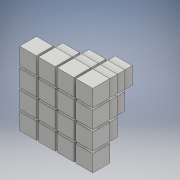
# Autodesk Inventor part: 方塊
Saved by Autodesk Inventor 2017 (Build 210142000, 142)
## iProperties
Created: 2021-05-20
Part Number: 方塊
Material: Generic
Document SubType Name: Modeling
Designer: user
Density: 1 g/cm^3
Appearance: Default
Author: user
Autodesk Inventor part; units mm, degrees
ref_plane "YZ Plane" through (0, 0, 0) normal (1, 0, 0) x (0, 1, 0)
ref_plane "XZ Plane" through (0, 0, 0) normal (0, 1, 0) x (-1, 0, 0)
ref_plane "XY Plane" through (0, 0, 0) normal (0, 0, 1) x (1, 0, 0)
sketch "Sketch1" plane through (0, 0, 0) normal (0, 1, 0) x (-1, 0, 0)
  line L0 (0, 0) -> (90, 0)
  line L1 (90, 0) -> (90, -90)
  line L2 (90, -90) -> (0, -90)
  line L3 (0, -90) -> (0, 0)
  dimension "d0" = 90
  dimension "d1" = 90
  constraints: 8 end point, 2 parallel, 1 horizontal, 1 perpendicular
  measures "d0" distance of L0.start L0.end
  measures "d1" distance of L2.end L0.start
extrude "Extrusion1" add sketch "Sketch1" along normal blind 90
pattern_linear "Rectangular Pattern1" count 4 spacing 100 along (0, 0, -1) count 4 spacing 100 along (1, 0, 0)
sketch "Sketch2" plane through (0, 90, 0) normal (0, 1, 0) x (1, 0, 0)
  line L0 (-40, 50) -> (50, 50)
  line L1 (50, 50) -> (50, 140)
  line L2 (50, 140) -> (-40, 140)
  line L3 (-40, 140) -> (-40, 50)
  line L4 (10, 100) -> (100, 100) projected
  line L5 (0, 0) -> (0, 90) projected
  line L6 (10, 100) -> (0, 90)
  point P0 (5, 95)
  dimension "d10" = 45
  dimension "d11" = 45
  dimension "d12" = 90
  dimension "d13" = 90
  constraints: 10 end point, 2 parallel, 1 horizontal, 1 midpoint, 1 perpendicular
  measures "d10" distance from line of L3 point (5, 95)
  measures "d11" distance from line of L0 point (5, 95)
  measures "d12" distance of L1.end L2.end
  measures "d13" distance of L2.end L0.start
extrude "Extrusion2" add sketch "Sketch2" along normal blind 90 separate body
pattern_linear "Rectangular Pattern2" count 3 spacing 100 along (1, 0, 0) count 3 spacing 100 along (0, 0, -1) bodies 2
sketch "Sketch3" plane through (0, 180, 0) normal (0, 1, 0) x (1, 0, 0)
  line L0 (10, 100) -> (100, 100) projected
  line L1 (100, 100) -> (100, 190) projected
  line L2 (100, 190) -> (10, 190) projected
  line L3 (10, 190) -> (10, 100) projected
  point P0 (0, 0)
extrude "Extrusion3" add sketch "Sketch3" along normal blind 90 separate body
pattern_linear "Rectangular Pattern3" count 2 spacing 100 along (0, 0, -1) count 2 spacing 100 along (1, 0, 0) bodies 3
sketch "Sketch4" plane through (10, 270, -200) normal (0, 1, 0) x (1, 0, 0)
  line L0 (50, -50) -> (140, -50) projected
  line L1 (140, -50) -> (140, 40) projected
  line L2 (140, 40) -> (50, 40) projected
  line L3 (50, 40) -> (50, -50) projected
  point P0 (-10, -200)
extrude "Extrusion4" add sketch "Sketch4" along normal blind 90 separate body
body "Solid1"
body "Solid2"
body "Solid3"
body "Solid4"
body "Solid5"
body "Solid6"
body "Solid7"
body "Solid8"
body "Solid9"
body "Solid10"
body "Solid11"
body "Solid12"
body "Solid13"
body "Solid14"
body "Solid15"
body "Solid16"
body "Solid17"
body "Solid18"
body "Solid19"
body "Solid20"
body "Solid21"
body "Solid22"
body "Solid23"
body "Solid24"
body "Solid25"
body "Solid26"
body "Solid27"
body "Solid28"
body "Solid29"
body "Solid30"
